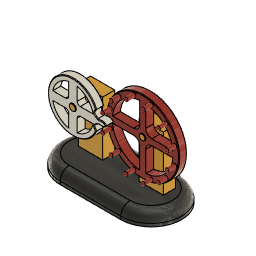
mech_wheels (Autodesk Fusion 360 design; units mm, degrees)
Autodesk Fusion 360 part; units mm, degrees
sketch "holder base" plane through (0, 0, 0) normal (0, 0, 1) x (1, 0, 0) in component "holder base"
  line L0 (0, 0) -> (100, 0)
  line L1 (100, 0) -> (100, -50)
  line L2 (100, -50) -> (0, -50)
  line L3 (0, -50) -> (0, 0)
  line L4 (15, -15) -> (35, -15)
  line L5 (35, -15) -> (35, -25)
  line L6 (35, -25) -> (15, -25)
  line L7 (15, -25) -> (15, -15)
  line L8 (85, -15) -> (65, -15)
  line L9 (65, -15) -> (65, -25)
  line L10 (65, -25) -> (85, -25)
  line L11 (85, -25) -> (85, -15)
  dimension "d1" = 100
  dimension "d2" = 50
  constraint horizontal L0
  constraint vertical L1
  constraint horizontal L2
  constraint vertical L3
  constraint coincident L0.start L3.end
  constraint horizontal L4
  constraint vertical L5
  constraint horizontal L6
  constraint vertical L7
  constraint horizontal L8
  constraint vertical L9
  constraint horizontal L10
  constraint vertical L11
  measures "d1" distance of L0.start L0.end
  measures "d2" distance of L0.start L2.end
extrude "Extrude1" add sketch "holder base" along normal blind 10 contours L0 L1 L2 L3 | L4 L5 L6 L7 | L8 L9 L10 L11 makes body 1 in component "holder base"
sketch "crank holder" plane through (0, 0, 10) normal (0, 0, 1) x (-1, 0, 0) in component "crank holder"
  line L0 (0, 50) -> (-100, 50)
  line L1 (-100, 50) -> (-100, 0)
  line L2 (-100, 0) -> (0, 0)
  line L3 (0, 0) -> (0, 50)
  line L4 (-15, 15) -> (-35, 15)
  line L5 (-35, 15) -> (-35, 25)
  line L6 (-35, 25) -> (-15, 25)
  line L7 (-15, 25) -> (-15, 15)
  constraint horizontal L4
  constraint vertical L5
  constraint horizontal L6
  constraint vertical L7
extrude "Extrude2" cut sketch "holder base" along normal blind 20 contours L4 L5 L6 L7 | L8 L9 L10 L11 bodies 1 in component "holder base"
extrude "Extrude1'" add sketch "crank holder" along normal blind -10 and the other way blind -45 separate body contours L4 L5 L6 L7 makes body 2 in component "crank holder"
sketch "wheel holder" plane through (0, 0, 0) normal (0, 0, 1) x (1, 0, 0) in component "wheel holder"
  line L0 (65, -15) -> (85, -15)
  line L1 (85, -15) -> (85, -25)
  line L2 (85, -25) -> (65, -25)
  line L3 (65, -25) -> (65, -15)
  constraint horizontal L0
  constraint vertical L1
  constraint horizontal L2
  constraint vertical L3
extrude "Extrude1''" add sketch "holder base" along normal blind 55 separate body contours L8 L9 L10 L11 makes body 3 in component "wheel holder"
sketch "wheel holder pin" plane through (0, -25, 0) normal (0, -1, 0) x (1, 0, 0) in component "wheel holder"
  line L0 (65, 0) -> (85, 0)
  line L1 (85, 0) -> (85, 55)
  line L2 (85, 55) -> (65, 55)
  line L3 (65, 55) -> (65, 0)
  circle A0 centre (75, 50) radius 2.5
  dimension "d13" = 5
  measures "d13" diameter of A0
sketch "crank holder pin" plane through (0, -25, 0) normal (0, -1, 0) x (1, 0, 0) in component "crank holder"
  line L0 (15, 55) -> (15, 0)
  line L1 (15, 0) -> (35, 0)
  line L2 (35, 0) -> (35, 55)
  line L3 (35, 55) -> (15, 55)
  line L4 (25, 55) -> (25, 52.5)
  circle A0 centre (25, 50) radius 2.5
  circle A1 centre (25, 50) radius 2.5
  dimension "d16" = 2.5
  constraint midpoint L3 L4.start
  constraint perpendicular L3 L4
  constraint coincident L4.end A0
  constraint concentric A0 A1
  measures "d16" distance of L4.start L4.end
extrude "Extrude2'" add sketch "crank holder pin" along normal blind 15 contours A0 A1 bodies 2 in component "crank holder"
extrude "Extrude3" add sketch "wheel holder pin" along normal blind 7.5 contours A0 bodies 3 in component "wheel holder"
sketch "wheel" plane through (0, -25, 0) normal (0, -1, 0) x (1, 0, 0) in component "wheel"
  circle A0 centre (75, 50) radius 30
  circle A1 centre (75, 50) radius 27.5
  circle A2 centre (75, 50) radius 2.5
  line L0 (75, 50) -> (45, 50) construction
  circle A3 centre (47.5, 50) radius 1.5
  dimension "d21" = 55
  dimension "d22" = 5
  constraint concentric A0 A1
  constraint concentric A0 A2
  constraint coincident A0.centre A1.centre
  constraint coincident A0 L0.end
  constraint horizontal L0
  constraint coincident A1 A3.centre
  constraint coincident L0 A3.centre
  measures "d21" diameter of A1
  measures "d22" diameter of A2
extrude "Extrude1'''" add sketch "wheel" along normal blind 7 and the other way blind -0.5 separate body contours A0 | A1 A3 | A1 A3 | A1 A3 makes body 4 in component "wheel"
extrude "Extrude2''" add sketch "wheel" along normal blind 15 and the other way blind -7 contours A1 A3 | A1 A3 picked at (48.003, 50) picked at (47.003, 50) bodies 4 in component "wheel"
pattern_circular "C-Pattern1" count 12 over 360 about axis through (75, -25, 50) along (0, -1, 0) of "Extrude2''" in component "wheel"
move_face "OffsetFaces1" offset -0.2 1 faces at (77.4876, -30, 49.7511) on bodies 3 in component "wheel holder"
sketch "crank" plane through (0, -25, 0) normal (0, -1, 0) x (1, 0, 0) in component "crank"
  circle A0 centre (25, 50) radius 2.5
  line L0 (15, 55) -> (15, 0)
  line L1 (15, 0) -> (35, 0)
  line L2 (35, 0) -> (35, 55)
  line L3 (35, 55) -> (15, 55)
  line L4 (25, 50) -> (65, 50) construction
  spline S0 degree 5 poles (45.5, 48) (45.6189, 48.0856) (45.8499, 48.2329) (46.1757, 48.3816) (46.5747, 48.447) (47.0474, 48.372) (47.5334, 48.2234) (48.0663, 48.0845) (48.6636, 48.0226) (49.3112, 48.0674) (49.9689, 48.2144) (50.5858, 48.4389) (51.1114, 48.7061) (51.5087, 48.9821) (51.7669, 49.2438) (51.917, 49.4908) (51.9918, 49.6868) (52.0444, 49.84) (52.0812, 49.946) (52.1, 50) knots 0 0 0 0 0 0 0.066667 0.133333 0.2 0.266667 0.333333 0.4 0.466667 0.533333 0.6 0.666667 0.733333 0.8 0.866667 0.933333 1 1 1 1 1 1
  line L5 (51.891, 49.4) -> (52.309, 50.6)
  spline S1 degree 5 poles (45.5, 52) (45.6189, 51.9144) (45.8499, 51.7671) (46.1757, 51.6184) (46.5747, 51.553) (47.0474, 51.628) (47.5334, 51.7766) (48.0663, 51.9155) (48.6636, 51.9774) (49.3112, 51.9326) (49.9689, 51.7856) (50.5858, 51.5611) (51.1114, 51.2939) (51.5087, 51.0179) (51.7669, 50.7562) (51.917, 50.5092) (51.9918, 50.3132) (52.0444, 50.16) (52.0812, 50.054) (52.1, 50) knots 0 0 0 0 0 0 0.066667 0.133333 0.2 0.266667 0.333333 0.4 0.466667 0.533333 0.6 0.666667 0.733333 0.8 0.866667 0.933333 1 1 1 1 1 1
  line L6 (44.7969, 47.4938) -> (46.2031, 48.5062)
  line L7 (44.7969, 52.5062) -> (46.2031, 51.4938)
  line L8 (51.891, 50.6) -> (52.309, 49.4)
  spline S2 degree 5 poles (45.5, 52) (45.1987, 52.1407) (44.6529, 52.4141) (44.0048, 52.8) (43.4413, 53.2599) (43.0238, 53.7161) (42.7213, 54.0832) (42.4299, 54.4251) (42.4313, 55.0275) (42.9524, 56.0394) (43.7354, 57.2175) (44.4298, 58.2478) (44.7058, 58.8885) (44.4203, 59.1055) (43.9332, 59.4358) (43.4152, 59.9749) (43.0161, 60.4634) (42.7198, 60.766) (42.5206, 60.9226) (42.4206, 60.9897) knots 0 0 0 0 0 0 0.066667 0.133333 0.2 0.266667 0.333333 0.4 0.466667 0.533333 0.6 0.666667 0.733333 0.8 0.866667 0.933333 1 1 1 1 1 1
  line L9 (44.8001, 58.5992) -> (44.2, 59.4)
  line L10 (42.6469, 53.8802) -> (42.3531, 55.1198)
  spline S3 degree 5 poles (45.5, 48) (45.1987, 47.8593) (44.6529, 47.5859) (44.0048, 47.2) (43.4413, 46.7401) (43.0238, 46.2839) (42.7213, 45.9168) (42.4299, 45.5749) (42.4313, 44.9725) (42.9524, 43.9606) (43.7354, 42.7825) (44.4298, 41.7522) (44.7058, 41.1115) (44.4203, 40.8945) (43.9332, 40.5642) (43.4152, 40.0251) (43.0161, 39.5366) (42.7198, 39.234) (42.5206, 39.0774) (42.4206, 39.0103) knots 0 0 0 0 0 0 0.066667 0.133333 0.2 0.266667 0.333333 0.4 0.466667 0.533333 0.6 0.666667 0.733333 0.8 0.866667 0.933333 1 1 1 1 1 1
  line L11 (47.6934, 50.9759) -> (43.3066, 53.0241)
  line L12 (43.3, 60.4) -> (41.5412, 61.5794)
  line L13 (47.6934, 49.0241) -> (43.3066, 46.9759)
  line L14 (42.6469, 46.1198) -> (42.3531, 44.8802)
  line L15 (44.8001, 41.4008) -> (44.2, 40.6)
  line L16 (43.3, 39.6) -> (41.5412, 38.4206)
  arc A1 (44.0836, 57.7503) -> (44.0836, 42.2497) centre (25, 50) ccw
  point P0 (48.2682, 48.0762)
  point P1 (51.5, 49)
  point P2 (48.2682, 51.9238)
  point P3 (51.5, 51)
  point P4 (42.5, 54.5)
  point P5 (44.5, 58.9996)
  point P6 (42.5, 45.5)
  point P7 (44.5, 41.0004)
  constraint concentric A0 A1
  constraint coincident A0.centre L4.start
  constraint horizontal L4
  constraint coincident L4 S0.end
  constraint midpoint S0.end L5
  constraint midpoint S0.start L6
  constraint symmetric L4 S0.start S1.start
  constraint symmetric L4 P0 P2
  constraint symmetric L4 P1 P3
  constraint symmetric L4 S0.end S1.end
  constraint symmetric L4 L5.start L8.start
  constraint symmetric L4 L5.end L8.end
  constraint symmetric L4 L6.start L7.start
  constraint symmetric L4 L6.end L7.end
  constraint coincident S2.end A1
  constraint midpoint P5 L9
  constraint midpoint P4 L10
  constraint midpoint S1.start L11
  constraint midpoint S2.end L12
  constraint symmetric L4 S1.start S0.start
  constraint symmetric L4 P4 P6
  constraint symmetric L4 P5 P7
  constraint symmetric L4 S2.end S3.end
  constraint symmetric L4 L9.start L15.start
  constraint symmetric L4 L9.end L15.end
  constraint symmetric L4 L10.start L14.start
  constraint symmetric L4 L10.end L14.end
  constraint symmetric L4 L11.start L13.start
  constraint symmetric L4 L11.end L13.end
  constraint symmetric L4 L12.start L16.start
  constraint symmetric L4 L12.end L16.end
  constraint coincident S2 A1.start
  constraint coincident S3 A1.end
extrude "Extrude4" add sketch "crank" along normal blind 6.5 separate body contours L0 L2 L3 A1 | L0 L2 L3 S0 S1 S2 S3 A1 makes body 5 in component "crank"
move_body "Move3" bodies 5 to x (1, 0, 0) y (0, 1, 0) z (0, 0, 1) at (0, -8, 0) in component "crank"
move_face "OffsetFaces2" offset -0.3 1 faces at (27.4876, -37.3333, 49.7511) on bodies 5 in component "crank"
fillet "Fillet1" radius 0.5 1 edges at (47.0302, -32, 39.1515) on bodies 4 in component "wheel"
fillet "Fillet2" radius 0.5 1 edges at (47.0302, -25.5, 39.1515) on bodies 4 in component "wheel"
fillet "Fillet1'" radius 0.49 14 edges at (4.4027, -39.5, 50) (4.4027, -33, 50) (42.6506, -39.5, 54.1818) (42.6506, -39.5, 54.1818) (42.6506, -33, 54.1818) (42.6506, -33, 54.1818) (42.6506, -39.5, 45.8182) (42.6506, -39.5, 45.8182) (42.6506, -33, 45.8182) (42.6506, -33, 45.8182) (49.6381, -39.5, 48.1521) (49.6381, -39.5, 51.8479) (49.6381, -33, 51.8479) (49.6381, -33, 48.1521) on bodies 5 in component "crank"
fillet "Fillet3" radius 1.5 12 edges at (49.702, -40, 63.9795) (46.1015, -40, 49.4576) (50.2444, -40, 35.081) (61.0205, -40, 24.702) (75.5424, -40, 21.1015) (89.919, -40, 25.2444) (100.298, -40, 36.0205) (103.8985, -40, 50.5424) (99.7556, -40, 64.919) (88.9795, -40, 75.298) (74.4576, -40, 78.8985) (60.081, -40, 74.7556) on bodies 4 in component "wheel"
fillet "Fillet1''" radius 25 4 edges at (100, 0, 5) (100, -50, 5) (0, 0, 5) (0, -50, 5) on bodies 1 in component "holder base"
fillet "Fillet2'" radius 7.5 4 edges at (0, -25, 10) (50, -50, 10) (100, -25, 10) (50, 0, 10) on bodies 1 in component "holder base"
sketch "wheel - cut" plane through (0, -32, 0) normal (0, -1, 0) x (1, 0, 0)
  circle A0 centre (75, 50) radius 2.5
  circle A1 centre (48.437, 42.8825) radius 1.5
  circle A2 centre (55.5546, 30.5546) radius 1.5
  circle A3 centre (67.8825, 23.437) radius 1.5
  circle A4 centre (82.1175, 23.437) radius 1.5
  circle A5 centre (94.4454, 30.5546) radius 1.5
  circle A6 centre (101.563, 42.8825) radius 1.5
  circle A7 centre (101.563, 57.1175) radius 1.5
  circle A8 centre (94.4454, 69.4454) radius 1.5
  circle A9 centre (82.1175, 76.563) radius 1.5
  circle A10 centre (67.8825, 76.563) radius 1.5
  circle A11 centre (55.5546, 69.4454) radius 1.5
  circle A12 centre (48.437, 57.1175) radius 1.5
  circle A13 centre (75, 50) radius 29.5
  circle A14 centre (75, 50) radius 25
  line L0 (75, 50) -> (75, 52.5) construction
  line L1 (75, 50) -> (72.5, 50) construction
  line L2 (72.5, 52.5) -> (77.5, 52.5) construction
  line L3 (77.5, 52.5) -> (77.5, 47.5) construction
  line L4 (77.5, 47.5) -> (72.5, 47.5) construction
  line L5 (72.5, 47.5) -> (72.5, 52.5) construction
  circle A15 centre (75, 50) radius 3.5355 construction
  line L6 (77.5, 47.5) -> (72.5, 47.5)
  line L7 (72.5, 47.5) -> (72.5, 52.5)
  line L8 (72.5, 52.5) -> (77.5, 52.5)
  line L9 (77.5, 52.5) -> (77.5, 47.5)
  line L10 (77.5, 52.5) -> (99.8747, 52.5)
  line L11 (99.8747, 52.5) -> (99.8747, 47.5)
  line L12 (99.8747, 47.5) -> (77.5, 47.5)
  line L13 (77.5, 47.5) -> (77.5, 52.5)
  line L14 (77.5, 52.5) -> (72.5, 52.5)
  line L15 (72.5, 52.5) -> (72.5, 74.8747)
  line L16 (72.5, 74.8747) -> (77.5, 74.8747)
  line L17 (77.5, 74.8747) -> (77.5, 52.5)
  line L18 (77.5, 47.5) -> (72.5, 47.5)
  line L19 (72.5, 47.5) -> (72.5, 25.1253)
  line L20 (72.5, 25.1253) -> (77.5, 25.1253)
  line L21 (77.5, 25.1253) -> (77.5, 47.5)
  line L22 (72.5, 47.5) -> (50.1253, 47.5)
  line L23 (50.1253, 47.5) -> (50.1253, 52.5)
  line L24 (50.1253, 52.5) -> (72.5, 52.5)
  line L25 (72.5, 52.5) -> (72.5, 47.5)
  line L26 (75, 25.1253) -> (75, 74.8747) construction
  line L27 (99.8747, 50) -> (50.1253, 50) construction
  arc A16 (67.5, 52.5) -> (72.5, 57.5) centre (67.5, 57.5) ccw
  arc A17 (72.5, 42.5) -> (67.5, 47.5) centre (67.5, 42.5) ccw
  arc A18 (82.5, 47.5) -> (77.5, 42.5) centre (82.5, 42.5) ccw
  arc A19 (77.5, 57.5) -> (82.5007, 52.5) centre (82.5, 57.5) ccw
  dimension "d83" = 50
  dimension "d84" = 5
  dimension "d85" = 5
  dimension "d86" = 5
  constraint concentric A0 A14
  constraint coincident A0.centre A13.centre
  constraint coincident A0 L0.end
  constraint vertical L0
  constraint coincident A0 L1.end
  constraint perpendicular L0 L1
  constraint horizontal L2
  constraint vertical L3
  constraint horizontal L4
  constraint vertical L5
  constraint coincident L4.end A15
  constraint coincident L2.end A15
  constraint horizontal L6
  constraint vertical L7
  constraint horizontal L8
  constraint vertical L9
  constraint horizontal L10
  constraint vertical L11
  constraint horizontal L12
  constraint vertical L13
  constraint coincident A14 L11.end
  constraint horizontal L14
  constraint vertical L15
  constraint horizontal L16
  constraint vertical L17
  constraint coincident A14 L15.end
  constraint horizontal L18
  constraint vertical L19
  constraint horizontal L20
  constraint vertical L21
  constraint coincident A14 L19.end
  constraint horizontal L22
  constraint vertical L23
  constraint horizontal L24
  constraint vertical L25
  constraint coincident A14 L23.end
  constraint tangent L22 A17
  constraint midpoint L20 L26.start
  constraint midpoint L16 L26.end
  constraint midpoint L11 L27.start
  constraint midpoint L23 L27.end
  constraint symmetric L27 A16 A17
  constraint symmetric L26 A17 A18
  constraint symmetric L26 A16 A19
  constraint coincident L15 A16.end
  constraint coincident L24 A16.start
  constraint coincident L22 A17.end
  constraint coincident L19 A17.start
  constraint coincident L21 A18.end
  constraint coincident L12 A18.start
  constraint coincident L10 A19.end
  constraint coincident L17 A19.start
  measures "d83" diameter of A14
  measures "d84" distance of L2.end L2.start
  measures "d85" distance of L3.end L4.end
  measures "d86" distance of L4.end L2.start
extrude "Extrude3'" cut sketch "wheel - cut" against normal blind 6.5 contours A14 L10 L17 A19 | A14 L12 L21 A18 | A14 L15 L24 A16 | A14 L19 L22 A17 sketch seen with x (0.965926, 0, -0.258819) y (0, 1, 0) z (0.258819, 0, 0.965926) at (-10.3854, 0, 21.1151) bodies 4 in component "wheel"
sketch "crank - cut" plane through (0, -39.5, 0) normal (0, -1, 0) x (1, 0, 0)
  circle A0 centre (25, 50) radius 2.8
  spline S0 degree 3 poles (43.5329, 57.7998) (43.3998, 57.595) (43.2648, 57.3915) (42.9342, 56.8847) (42.74, 56.581) (42.4281, 56.0402) (42.3031, 55.8071) (42.1263, 55.3932) (42.0638, 55.2167) (41.9897, 54.8617) (41.9767, 54.6831) (42.019, 54.374) (42.0594, 54.2427) (42.1557, 54.0444) (42.1999, 53.9717) (42.2483, 53.9021) (42.3911, 53.6968) (42.5584, 53.5099) (42.904, 53.1289) (43.0928, 52.9429) (43.6083, 52.5048) (43.9524, 52.2722) (44.6164, 51.886) (44.9309, 51.726) (45.2521, 51.575) knots -0.824406 -0.824406 -0.824406 -0.824406 -0.751128 -0.751128 -0.642879 -0.642879 -0.563765 -0.563765 -0.507857 -0.507857 -0.454952 -0.454952 -0.414255 -0.414255 -0.38882 -0.38882 -0.38882 -0.3138 -0.3138 -0.234492 -0.234492 -0.111029 -0.111029 -0.004481 -0.004481 -0.004481 -0.004481
  arc A1 (43.5329, 57.7998) -> (43.5329, 42.2002) centre (25, 50) ccw
  spline S1 degree 3 poles (45.2521, 48.425) (44.9309, 48.274) (44.6164, 48.114) (43.9524, 47.7278) (43.6083, 47.4952) (43.0928, 47.0571) (42.904, 46.8711) (42.5584, 46.4901) (42.3911, 46.3032) (42.2483, 46.0979) (42.1999, 46.0283) (42.1557, 45.9556) (42.0594, 45.7573) (42.019, 45.626) (41.9767, 45.3169) (41.9897, 45.1383) (42.0638, 44.7833) (42.1263, 44.6068) (42.3031, 44.1929) (42.4281, 43.9598) (42.74, 43.419) (42.9342, 43.1153) (43.2648, 42.6085) (43.3998, 42.405) (43.5329, 42.2002) knots -0.845233 -0.845233 -0.845233 -0.845233 -0.738686 -0.738686 -0.615223 -0.615223 -0.535915 -0.535915 -0.460895 -0.460895 -0.460895 -0.43546 -0.43546 -0.394763 -0.394763 -0.341858 -0.341858 -0.28595 -0.28595 -0.206836 -0.206836 -0.098587 -0.098587 -0.025309 -0.025309 -0.025309 -0.025309
  spline S2 degree 3 poles (51.5812, 50) (51.5738, 49.9788) (51.5662, 49.9575) (51.5179, 49.8231) (51.4738, 49.7098) (51.2932, 49.4465) (51.1317, 49.3227) (50.7484, 49.0718) (50.5144, 48.9568) (50.034, 48.7636) (49.7863, 48.6863) (49.5332, 48.6308) (49.3015, 48.58) (49.065, 48.5478) (48.5907, 48.5329) (48.3532, 48.5516) (47.8562, 48.6426) (47.5994, 48.7217) (46.9906, 48.8778) (46.625, 48.9309) (45.9553, 48.8185) (45.6596, 48.6879) (45.3443, 48.4882) (45.2978, 48.457) (45.2521, 48.425) knots -0.705906 -0.705906 -0.705906 -0.705906 -0.699166 -0.699166 -0.663075 -0.663075 -0.603381 -0.603381 -0.525647 -0.525647 -0.447914 -0.447914 -0.447914 -0.37676 -0.37676 -0.305605 -0.305605 -0.225188 -0.225188 -0.116589 -0.116589 -0.021438 -0.021438 -0.004715 -0.004715 -0.004715 -0.004715
  spline S3 degree 3 poles (45.2521, 51.575) (45.2978, 51.543) (45.3443, 51.5118) (45.6596, 51.3121) (45.9553, 51.1815) (46.625, 51.0691) (46.9906, 51.1222) (47.5994, 51.2783) (47.8562, 51.3574) (48.3532, 51.4484) (48.5907, 51.4671) (49.065, 51.4522) (49.3015, 51.42) (49.5332, 51.3692) (49.7863, 51.3137) (50.034, 51.2364) (50.5144, 51.0432) (50.7484, 50.9282) (51.1317, 50.6773) (51.2932, 50.5535) (51.4738, 50.2902) (51.5179, 50.1769) (51.5662, 50.0425) (51.5738, 50.0212) (51.5812, 50) knots -0.718274 -0.718274 -0.718274 -0.718274 -0.701551 -0.701551 -0.6064 -0.6064 -0.497801 -0.497801 -0.417384 -0.417384 -0.346229 -0.346229 -0.275075 -0.275075 -0.275075 -0.197342 -0.197342 -0.119608 -0.119608 -0.059914 -0.059914 -0.023822 -0.023822 -0.017083 -0.017083 -0.017083 -0.017083
  circle A2 centre (25, 50) radius 17
  spline S4 degree 5 poles (25, 67) (26.3986, 67) (29.0047, 66.8264) (32.3407, 66.0454) (35.6978, 64.0156) (38.3555, 60.133) (39.7817, 55.3081) (40.2218, 50) (39.7817, 44.6919) (38.3555, 39.867) (35.6978, 35.9844) (32.3407, 33.9546) (29.0047, 33.1736) (26.3986, 33) (25, 33) knots 0 0 0 0 0 0 0.1 0.2 0.3 0.4 0.5 0.6 0.7 0.8 0.9 1 1 1 1 1 1
  line L0 (30, 33) -> (20, 33)
  line L1 (20, 67) -> (30, 67)
  circle A3 centre (25, 50) radius 2.8
  circle A4 centre (25, 50) radius 3.5
  line L2 (25, 50) -> (21.5, 50) construction
  line L3 (25, 50) -> (25, 53.5) construction
  line L4 (25, 53.5) -> (21.5, 53.5) construction
  line L5 (21.5, 50) -> (21.5, 53.5) construction
  line L6 (25, 53.5) -> (8.3652, 53.5)
  line L7 (8.3652, 53.5) -> (8.3652, 46.4952)
  line L8 (8.3652, 46.4952) -> (25, 46.4952)
  line L9 (25, 46.4952) -> (25, 53.5)
  line L10 (21.5, 53.5) -> (28.5, 53.5)
  line L11 (28.5, 53.5) -> (28.5, 33.2524)
  line L12 (28.5, 33.2524) -> (21.5, 33.2524)
  line L13 (21.5, 33.2524) -> (21.5, 53.5)
  line L14 (21.5, 46.4952) -> (39.7934, 46.4952)
  line L15 (39.7934, 46.4952) -> (39.7934, 53.5)
  line L16 (39.7934, 53.5) -> (21.5, 53.5)
  line L17 (21.5, 53.5) -> (21.5, 46.4952)
  line L18 (28.5, 46.4952) -> (21.5, 46.4952)
  line L19 (21.5, 46.4952) -> (21.5, 66.6358)
  line L20 (21.5, 66.6358) -> (28.5, 66.6358)
  line L21 (28.5, 66.6358) -> (28.5, 46.4952)
  line L22 (8, 49.9976) -> (42, 49.9976) construction
  arc A5 (28.5, 56) -> (31.0005, 53.5) centre (31, 56) ccw
  arc A6 (19, 53.5) -> (21.5, 56) centre (19, 56) ccw
  arc A7 (21.5, 43.9952) -> (19, 46.4952) centre (19, 43.9952) ccw
  arc A8 (31.0005, 46.4952) -> (28.5, 43.9952) centre (31, 43.9952) ccw
  line L23 (39.7934, 53.5) -> (41.6358, 53.5)
  line L24 (39.7934, 46.4952) -> (41.6348, 46.4952)
  line L25 (8.3652, 53.5) -> (8.3609, 53.4843)
  point P0 (40, 50)
  dimension "d89" = 7
  dimension "d90" = 7
  constraint concentric A0 A2
  constraint coincident A2 S4.start
  constraint coincident A2 S4.end
  constraint midpoint S4.end L0
  constraint tangent A2 L0
  constraint midpoint S4.start L1
  constraint tangent A2 L1
  constraint concentric A2 A3
  constraint concentric A2 A4
  constraint coincident A0.centre A1.centre
  constraint coincident A4 L2.end
  constraint horizontal L2
  constraint coincident A4 L3.end
  constraint perpendicular L2 L3
  constraint tangent A4 L4
  constraint horizontal L6
  constraint vertical L7
  constraint horizontal L8
  constraint vertical L9
  constraint coincident A2 L7.end
  constraint horizontal L10
  constraint vertical L11
  constraint horizontal L12
  constraint vertical L13
  constraint coincident S4 L11.end
  constraint horizontal L14
  constraint vertical L15
  constraint horizontal L16
  constraint vertical L17
  constraint coincident S4 L15.end
  constraint coincident L8 L14.start
  constraint coincident L13 L14.start
  constraint horizontal L18
  constraint vertical L19
  constraint horizontal L20
  constraint vertical L21
  constraint coincident A2 L19.end
  constraint coincident L11 L18.start
  constraint coincident L14 L18.start
  constraint tangent L21 A5
  constraint tangent L19 A6
  constraint coincident A2 L22.start
  constraint coincident A2 L22.end
  constraint parallel L2 L22
  constraint symmetric L22 A5 A8
  constraint symmetric L22 A6 A7
  constraint coincident L16 A5.end
  constraint coincident L21 A5.start
  constraint coincident L19 A6.end
  constraint coincident L6 A6.start
  constraint coincident L8 A7.end
  constraint coincident L13 A7.start
  constraint coincident L11 A8.end
  constraint coincident L14 A8.start
  constraint coincident A2 L23.end
  constraint perpendicular L15 L23
  constraint coincident A2 L24.end
  constraint perpendicular L15 L24
  constraint coincident A2 L25.end
  measures "d89" diameter of A4
  measures "d90" distance of L4.end L10.end
extrude "Extrude6" cut sketch "crank - cut" against normal blind 6.5 contours A2 S4 L11 L14 A8 | A2 L6 L19 A6 L25 | A2 S4 L16 L21 A5 | A2 L8 L13 A7 | A2 S4 L23 | A2 S4 L14 L24 bodies 5 in component "crank"
component "holder base" placed x (1, 0, 0) y (0, 1, 0) z (0, 0, 1) at (0, 0, 0)
component "crank holder" placed x (1, 0, 0) y (0, 1, 0) z (0, 0, 1) at (0, 0, 0)
component "wheel holder" placed x (1, 0, 0) y (0, 1, 0) z (0, 0, 1) at (0, 0, 0)
component "wheel" placed x (0.965926, 0, 0.258819) y (0, 1, 0) z (-0.258819, 0, 0.965926) at (15.4965, 0, -17.7077)
component "crank" placed x (1, 0, 0) y (0, 1, 0) z (0, 0, 1) at (0, 0, 0)
named bodies: "crank holder", "wheel holder", "wheel", "crank"
